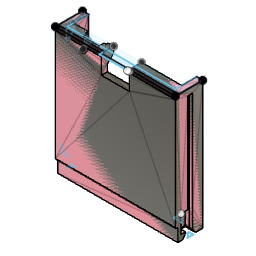
MicrocontrollerHousing (Autodesk Fusion 360 design; units mm, degrees)
Autodesk Fusion 360 part; units mm, degrees
sketch "Sketch1" plane through (0, 0, 0) normal (0, 0, 1) x (1, 0, 0)
ref_plane "WorkPlane1" through (0, 0, 0) normal (0, 0, 1) x (1, 0, 0)
sketch "Sketch2" plane through (0, 0, 0) normal (0, 0, 1) x (1, 0, 0)
  line L0 (-0.0018, 6.8149) -> (30, 6.8149)
  line L1 (30, 6.8149) -> (30, 0)
  line L2 (30, 0) -> (-0.0018, 0)
  line L3 (-0.0018, 0) -> (-0.0018, 6.8149)
  line L4 (14.9991, 3.4075) -> (25.7991, 3.4075)
  line L5 (14.9991, 3.4075) -> (4.1991, 3.4075)
  line L6 (14.9991, 4.3075) -> (4.6991, 4.3075)
  line L7 (14.9991, 4.3075) -> (25.2991, 4.3075)
  line L8 (14.9991, 2.5075) -> (4.6991, 2.5075)
  line L9 (14.9991, 2.5075) -> (25.2991, 2.5075)
  line L10 (14.9991, 4.3075) -> (25.2991, 4.3075)
  line L11 (14.9991, 4.3075) -> (4.6991, 4.3075)
  line L12 (25.7991, 3.8075) -> (25.7991, 3.4075)
  line L13 (4.1991, 3.0075) -> (4.1991, 3.4075)
  line L14 (4.1991, 3.8075) -> (4.1991, 3.4075)
  line L15 (25.7991, 3.4075) -> (25.7991, 3.0075)
  arc A0 (4.6991, 4.3075) -> (4.1991, 3.8075) centre (4.6991, 3.8075) ccw
  arc A1 (4.1991, 3.0075) -> (4.6991, 2.5075) centre (4.6991, 3.0075) ccw
  arc A2 (25.2991, 2.5075) -> (25.7991, 3.0075) centre (25.2991, 3.0075) ccw
  arc A3 (25.7991, 3.8075) -> (25.2991, 4.3075) centre (25.2991, 3.8075) ccw
  line L16 (14.9991, 3.4075) -> (14.9995, 3.4074)
  line L17 (15, 3.4075) -> (14.9995, 3.4074)
  dimension "d2" = 10.8
  dimension "d3" = 10.8
  dimension "d8" = 0.5
  constraint horizontal L0
  constraint vertical L1
  constraint horizontal L2
  constraint vertical L3
  constraint parallel L2 L4
  constraint parallel L4 L5
  constraint perpendicular L4 L12
  constraint perpendicular L5 L13
  constraint perpendicular L5 L14
  constraint parallel L5 L6
  constraint parallel L4 L7
  constraint tangent L14 A0
  constraint tangent L6 A0
  constraint parallel L5 L8
  constraint tangent L13 A1
  constraint tangent L8 A1
  constraint equal A0 A1
  constraint parallel L4 L9
  constraint tangent L9 A2
  constraint tangent L15 A2
  constraint equal A0 A2
  constraint tangent L12 A3
  constraint tangent L7 A3
  constraint equal A0 A3
  constraint parallel L4 L10
  constraint parallel L5 L11
  constraint coincident L4 L17.start
  measures "d2" distance of L4.start L4.end
  measures "d3" distance of L4.start L5.end
  measures "d8" radius of A0
sketch "Sketch4" plane through (0, 0, 0) normal (1, 0, 0) x (0, 1, 0)
  line L0 (6.8002, -0.0004) -> (6.8002, 32)
  line L1 (6.8002, 32) -> (0.8415, 32)
  line L2 (6.8002, -0.0004) -> (-0.2407, -0.0004)
  line L3 (-0.0066, 3.4989) -> (-0.0585, 31.0983)
  line L4 (4.9902, -0.0004) -> (4.2999, 0.9325)
  line L5 (4.2999, 0.9325) -> (4.25, 0.9325)
  line L6 (4.25, 0.9325) -> (4.25, 4.0597)
  line L7 (4.25, 4.0597) -> (2.5001, 4.0597)
  line L8 (2.5001, 1.39) -> (2.5001, 0.9325)
  line L9 (2.5001, 0.9325) -> (2.4506, 0.9325)
  line L10 (2.4506, 0.9325) -> (1.7589, -0.0004)
  line L11 (2.5001, 1.39) -> (1.4001, 1.39)
  line L12 (1.4001, 1.39) -> (1.4001, 5.86)
  line L13 (1.4001, 5.86) -> (3.0784, 5.86)
  line L14 (3.0784, 5.86) -> (3.0784, 30.5)
  line L15 (3.0784, 30.5) -> (4.25, 30.5)
  line L16 (4.25, 30.5) -> (4.25, 4.0597)
  line L17 (0.5999, -0.0004) -> (0.5999, 3.2)
  line L18 (0.5999, 3.2) -> (0.294, 3.1994)
  arc A0 (0.8415, 32) -> (-0.0585, 31.0983) centre (0.8415, 31.1) ccw
  arc A1 (-0.0066, 3.4989) -> (0.294, 3.1994) centre (0.2934, 3.4994) ccw
  line L19 (2.5001, 4.0597) -> (1.4001, 4.0597)
  dimension "d9" = 0.9
  dimension "d10" = 0.3
  constraint vertical L0
  constraint perpendicular L0 L1
  constraint perpendicular L0 L2
  constraint coincident L2 L4.start
  constraint parallel L2 L5
  constraint perpendicular L5 L6
  constraint perpendicular L6 L7
  constraint perpendicular L7 L8
  constraint perpendicular L8 L9
  constraint coincident L2 L10.end
  constraint perpendicular L8 L11
  constraint perpendicular L11 L12
  constraint perpendicular L12 L13
  constraint perpendicular L13 L14
  constraint perpendicular L14 L15
  constraint coincident L2 L17.start
  constraint perpendicular L2 L17
  constraint perpendicular L3 L18
  constraint tangent L1 A0
  constraint tangent L3 A0
  constraint tangent L18 A1
  constraint tangent L3 A1
  constraint coincident L12 L19.end
  constraint perpendicular L12 L19
  measures "d9" radius of A0
  measures "d10" radius of A1
ref_plane "WorkPlane2" through (14.9991, 3.4075, 32) normal (0, 0, 1) x (1, 0, 0)
sketch "Sketch5" plane through (14.9991, 3.4075, 32) normal (0, 0, 1) x (1, 0, 0)
  line L0 (-14.9991, 3.3927) -> (-14.9991, -3.4075)
  line L1 (-14.9991, -3.4075) -> (15.0009, -3.4075)
  line L2 (15.0009, -3.4075) -> (15.0009, 3.4075)
  line L3 (13.5009, 3.3927) -> (13.5009, 3.4067)
  line L4 (13.5009, 3.3927) -> (13.5009, -1.9074)
  line L5 (13.5009, -1.9074) -> (-13.4991, -1.9074)
  line L6 (-13.4991, -1.9074) -> (-13.5017, 3.3934)
  line L7 (15.0009, 3.4075) -> (13.5009, 3.4067)
  line L8 (-13.5017, 3.3934) -> (-14.9991, 3.3927)
  point P0 (-14.9991, 3.3927)
  point P1 (-14.9991, -3.4075)
  point P2 (15.0009, -3.4075)
  point P3 (15.0009, 3.4075)
  constraint coincident P0 L0.start
  constraint coincident P1 L0.end
  constraint coincident P2 L1.end
  constraint coincident P3 L2.end
  constraint perpendicular L3 L7
  constraint perpendicular L1 L4
  constraint perpendicular L4 L5
  constraint coincident L6.end L7
  constraint perpendicular L6 L7
  constraint collinear L7 L8
extrude "Extrude1" add sketch "Sketch5" against normal blind 32
extrude "Extrude2" add sketch "Sketch2" along normal blind 2
sketch "Side Slats" plane through (0, 0, 0) normal (0, 0, 1) x (1, 0, 0)
  line L0 (29.9999, 3.0777) -> (29.19, 3.93)
  line L1 (29.19, 3.93) -> (29.19, 4.25)
  line L2 (29.19, 4.25) -> (30, 4.25)
  line L3 (-0.0001, 3.0776) -> (0.81, 3.93)
  line L4 (0.81, 3.93) -> (0.81, 4.25)
  line L5 (0.81, 4.25) -> (0, 4.25)
  line L6 (-0.0001, 3.0776) -> (-0.201, 2.8662)
  line L7 (-0.201, 2.8662) -> (-0.2009, 4.25)
  line L8 (0, 4.25) -> (-0.2009, 4.25)
  line L9 (30, 4.25) -> (30.168, 4.25)
  line L10 (29.9999, 3.0777) -> (30.168, 2.9008)
  line L11 (30.168, 2.9008) -> (30.168, 4.25)
  constraint vertical L1
  constraint perpendicular L1 L2
  constraint vertical L4
  constraint perpendicular L4 L5
  constraint parallel L3 L6
  constraint perpendicular L7 L8
  constraint parallel L0 L10
  constraint perpendicular L9 L11
extrude "Extrude16" cut sketch "Side Slats" along normal blind 30.5
sketch "Sketch7" plane through (0, 0, 0) normal (1, 0, 0) x (0, 1, 0)
extrude "Extrude4" cut sketch "Sketch4" along normal blind 1.8 contours L2 L4 L5 L6 L7 L8 L9 L10 L11 L12 L19
extrude "Extrude5" cut sketch "Sketch4" against normal blind 1.2 contours L2 L4 L5 L6 L7 L8 L9 L10 L11 L12 L19
ref_plane "WorkPlane3" through (30, 0, 0) normal (1, 0, 0) x (0, 1, 0)
sketch "Sketch8" plane through (30, 0, 0) normal (1, 0, 0) x (0, 1, 0)
  line L0 (1.76, 0) -> (2.4501, 0.9324)
  line L1 (2.4501, 0.9324) -> (2.5001, 0.9324)
  line L2 (2.5001, 0.9324) -> (2.5001, 1.3897)
  line L3 (2.5001, 4.0595) -> (4.25, 4.0602)
  line L4 (4.25, 4.0602) -> (4.25, 0.9324)
  line L5 (4.25, 0.9324) -> (4.3, 0.9324)
  line L6 (4.3, 0.9324) -> (4.9902, -0.0001)
  line L7 (4.9902, -0.0001) -> (1.76, 0)
  line L8 (2.5001, 1.3897) -> (1.4001, 1.3897)
  line L9 (1.4001, 1.3897) -> (1.4001, 4.06)
  line L10 (1.4001, 4.06) -> (2.5001, 4.0595)
  constraint horizontal L1
  constraint perpendicular L1 L2
  constraint perpendicular L1 L4
  constraint perpendicular L4 L5
  constraint perpendicular L2 L8
  constraint perpendicular L8 L9
extrude "Extrude6" cut sketch "Sketch8" against normal blind 1.8
ref_plane "WorkPlane4" through (0, 0, 1.5) normal (0, 0, 1) x (1, 0, 0)
sketch "Sketch9" plane through (0, 0, 1.5) normal (0, 0, 1) x (1, 0, 0)
  line L0 (1.5, 5.3) -> (2.5, 5.3)
  line L1 (2.5, 5.3) -> (2.5, 1.5)
  line L2 (2.5, 1.5) -> (1.5, 1.5)
  line L3 (28.5, 5.3) -> (27.5, 5.3)
  line L4 (27.5, 5.3) -> (27.5, 1.5001)
  line L5 (27.5, 1.5001) -> (28.5, 1.5001)
  line L6 (1.6305, 5.3) -> (1.4386, 5.3)
  line L7 (1.4386, 5.3) -> (1.4386, 1.5)
  line L8 (1.4386, 1.5) -> (1.5958, 1.5)
  line L9 (28.4487, 5.3) -> (28.5452, 5.3)
  line L10 (28.5452, 5.3) -> (28.5453, 1.5001)
  line L11 (28.4238, 1.5001) -> (28.5453, 1.5001)
  constraint horizontal L0
  constraint perpendicular L0 L1
  constraint perpendicular L1 L2
  constraint horizontal L3
  constraint perpendicular L3 L4
  constraint perpendicular L4 L5
  constraint coincident L0 L6.start
  constraint parallel L0 L6
  constraint perpendicular L2 L7
  constraint coincident L2 L8.end
  constraint parallel L2 L8
  constraint coincident L3 L9.start
  constraint perpendicular L9 L10
  constraint coincident L5 L11.start
  constraint perpendicular L10 L11
extrude "Extrude7" add sketch "Sketch9" along normal blind 4 contours L0 L1 L2 L6 L7 L8
extrude "Extrude8" add sketch "Sketch9" along normal blind 4 contours L3 L4 L5 L9 L10 L11
ref_plane "WorkPlane5" through (0, 6, 0) normal (0, 1, 0) x (0, 0, 1)
sketch "Sketch10" plane through (0, 6, 0) normal (0, 1, 0) x (1, 0, 0)
  line L0 (2.5, -4.5) -> (1.5001, -5.5)
  line L1 (1.5001, -5.5) -> (2.5, -5.5)
  line L2 (2.5, -5.5) -> (2.5, -4.5)
  line L3 (28.5, -5.5) -> (27.5, -5.5)
  line L4 (27.5, -5.5) -> (27.5, -4.5)
  line L5 (27.5, -4.5) -> (28.5, -5.5)
  constraint horizontal L1
  constraint perpendicular L1 L2
  constraint perpendicular L2 L3
  constraint perpendicular L3 L4
extrude "Extrude9" cut sketch "Sketch10" against normal blind 4.5
extrude "Extrude10" cut sketch "Sketch8" against normal blind 1.8
extrude "Extrude11" cut sketch "Sketch4" along normal blind 1.8 contours L2 L4 L5 L6 L7 L8 L9 L10 L11 L12 L19
sketch "Sketch11" plane through (30, 0, 0) normal (1, 0, 0) x (0, 1, 0)
  line L0 (1.76, 0) -> (2.4501, 0.9324)
  line L1 (2.4501, 0.9324) -> (2.5001, 0.9324)
  line L2 (2.5001, 0.9324) -> (2.5001, 1.3897)
  line L3 (2.5001, 1.3897) -> (1.4001, 1.3897)
  line L4 (1.4001, 1.3897) -> (1.4001, 4.06)
  line L5 (1.4001, 4.06) -> (2.5001, 4.0595)
  line L6 (2.5001, 4.0595) -> (3.0776, 4.0597)
  line L7 (6.8149, 32) -> (0, 32)
  line L8 (0, 32) -> (0, 0)
  line L9 (4.9901, 0) -> (6.8149, 0)
  line L10 (0.6001, 0) -> (0.012, 0)
  line L11 (0.012, 3.1995) -> (0.6001, 3.1995)
  line L12 (0.6001, 3.1995) -> (0.6001, 0)
  line L13 (0.0679, 0) -> (-0.3097, 0)
  line L14 (-0.3097, 0) -> (-0.3097, 3.1995)
  line L15 (0.0854, 3.1995) -> (-0.3097, 3.1995)
  line L16 (0, 3.5529) -> (0, 3.1995)
  line L17 (0.6001, 3.1408) -> (0.6001, 3.6309)
  line L18 (0.6001, 3.6309) -> (0, 3.6309)
  line L19 (0, 3.5218) -> (0, 3.6309)
  line L20 (3.0776, 4.0597) -> (3.0776, 30.5)
  line L21 (3.0776, 30.5) -> (4.25, 30.5)
  line L22 (4.25, 30.5) -> (4.25, 0.9324)
  line L23 (4.25, 0.9324) -> (4.3, 0.9324)
  line L24 (4.3, 0.9324) -> (4.9901, 0)
  line L25 (6.8149, 0) -> (6.8149, 2)
  line L26 (6.8149, 2) -> (6.8149, 32)
  line L27 (0, 0) -> (1.76, 0)
  constraint horizontal L10
  constraint horizontal L11
  constraint vertical L12
  constraint coincident L9 L10.start
  constraint coincident L10 L13.start
  constraint perpendicular L13 L14
  constraint coincident L11 L15.start
  constraint perpendicular L14 L15
  constraint coincident L8 L16.start
  constraint coincident L15 L16.end
  constraint coincident L8 L16.end
  constraint perpendicular L15 L16
  constraint coincident L12 L17.start
  constraint perpendicular L11 L17
  constraint coincident L8 L18.end
  constraint perpendicular L8 L18
  constraint coincident L16 L19.start
extrude "Extrude12" cut sketch "Sketch11" against normal through all contours L8 L10 L11 L12 L13 L15 L17 L27 | L8 L13 L14 L15
sketch "Sketch12" plane through (30, 0, 0) normal (1, 0, 0) x (0, 1, 0)
  line L0 (0.6001, 3.1995) -> (0.6001, 0)
  line L1 (0.6001, 0) -> (1.76, 0)
  line L2 (1.76, 0) -> (2.4501, 0.9324)
  line L3 (2.4501, 0.9324) -> (2.5001, 0.9324)
  line L4 (2.5001, 0.9324) -> (2.5001, 1.3897)
  line L5 (2.5001, 1.3897) -> (1.4001, 1.3897)
  line L6 (1.4001, 1.3897) -> (1.4001, 4.06)
  line L7 (1.4001, 4.06) -> (2.5001, 4.0595)
  line L8 (2.5001, 4.0595) -> (3.0776, 4.0597)
  line L9 (6.8149, 32) -> (0, 32)
  line L10 (0, 32) -> (0, 3.1995)
  line L11 (0, 3.1995) -> (0.6001, 3.1995)
  line L12 (0, 3.4998) -> (0.716, 3.4998)
  line L13 (0.6001, 3.1995) -> (0.6001, 3.4998)
  line L14 (0, 3.4998) -> (0, 3.4995)
  line L15 (0.6001, 3.1995) -> (0.3, 3.1995)
  arc A0 (0, 3.4995) -> (0.3, 3.1995) centre (0.3, 3.4995) ccw
  line L16 (3.0776, 4.0597) -> (3.0776, 30.5)
  line L17 (3.0776, 30.5) -> (4.25, 30.5)
  line L18 (4.25, 30.5) -> (4.25, 0.9324)
  line L19 (4.25, 0.9324) -> (4.3, 0.9324)
  line L20 (4.3, 0.9324) -> (4.9901, 0)
  line L21 (4.9901, 0) -> (6.8149, 0)
  line L22 (6.8149, 0) -> (6.8149, 2)
  line L23 (6.8149, 2) -> (6.8149, 32)
  dimension "d37" = 0.3
  constraint coincident L10 L12.start
  constraint perpendicular L10 L12
  constraint coincident L0.start L11.end
  constraint coincident L12 L13.end
  constraint perpendicular L12 L13
  constraint tangent L15 A0
  constraint tangent L14 A0
  measures "d37" radius of A0
extrude "Extrude13" cut sketch "Sketch12" against normal through all contours L10 L11 A0
sketch "Sketch13" plane through (0, 0, 0) normal (0, 0, -1) x (1, 0, 0)
  line L0 (25.7991, -3.0075) -> (25.7991, -3.8075)
  arc A0 (25.2991, -4.3075) -> (25.7991, -3.8075) centre (25.2991, -3.8075) ccw
  line L1 (25.2991, -4.3075) -> (4.6991, -4.3075)
  arc A1 (4.1991, -3.8075) -> (4.6991, -4.3075) centre (4.6991, -3.8075) ccw
  line L2 (4.1991, -3.8075) -> (4.1991, -3.0075)
  arc A2 (4.6991, -2.5075) -> (4.1991, -3.0075) centre (4.6991, -3.0075) ccw
  line L3 (4.6991, -2.5075) -> (25.2991, -2.5075)
  arc A3 (25.7991, -3.0075) -> (25.2991, -2.5075) centre (25.2991, -3.0075) ccw
  line L4 (30, -0.6001) -> (-0.0018, -0.6001)
  line L5 (-0.0018, -0.6001) -> (-0.0018, -1.7592)
  line L6 (-0.0018, -1.7592) -> (1.8, -1.7592)
  line L7 (1.8, -1.7592) -> (1.8, -4.9899)
  line L8 (1.8, -4.9899) -> (-0.0018, -4.9899)
  line L9 (-0.0018, -4.9899) -> (-0.0018, -6.8149)
  line L10 (-0.0018, -6.8149) -> (30, -6.8149)
  line L11 (30, -6.8149) -> (30, -4.9901)
  line L12 (30, -4.9901) -> (28.2, -4.9901)
  line L13 (28.2, -4.9901) -> (28.2, -1.76)
  line L14 (28.2, -1.76) -> (30, -1.76)
  line L15 (30, -1.76) -> (30, -0.6001)
  line L16 (14.6109, -2.2) -> (17.9456, -2.2)
  line L17 (19.2456, -3.5) -> (19.2456, -3.5306)
  line L18 (17.9456, -4.8306) -> (14.6109, -4.8306)
  line L19 (14.6109, -2.2) -> (12.0539, -2.2)
  line L20 (10.7539, -3.5) -> (10.7539, -3.5306)
  line L21 (12.0539, -4.8306) -> (14.6109, -4.8306)
  arc A4 (12.0539, -2.2) -> (10.7539, -3.5) centre (12.0539, -3.5) ccw
  arc A5 (10.7539, -3.5306) -> (12.0539, -4.8306) centre (12.0539, -3.5306) ccw
  arc A6 (19.2456, -3.5) -> (17.9456, -2.2) centre (17.9456, -3.5) ccw
  arc A7 (17.9456, -4.8306) -> (19.2456, -3.5306) centre (17.9456, -3.5306) ccw
  dimension "d39" = 1.3
  dimension "d40" = 1.3
  dimension "d41" = 1.3
  dimension "d42" = 1.3
  constraint horizontal L16
  constraint vertical L17
  constraint horizontal L18
  constraint horizontal L19
  constraint vertical L20
  constraint horizontal L21
  constraint tangent L20 A4
  constraint tangent L19 A4
  constraint tangent L20 A5
  constraint tangent L21 A5
  constraint tangent L16 A6
  constraint tangent L17 A6
  constraint tangent L17 A7
  constraint tangent L18 A7
  measures "d39" radius of A4
  measures "d40" radius of A5
  measures "d41" radius of A6
  measures "d42" radius of A7
extrude "Extrude14" add sketch "Sketch13" against normal blind 2 contours L0 A0 L1 L3 A3 L17 A6 A7 | L1 L3 L17 L20 A4 A5 A6 A7 | L1 A1 L2 A2 L3 L20 A4 A5
extrude "Extrude15" cut sketch "Sketch13" against normal through all contours L1 L3 L17 L20 A4 A5 A6 A7 | L3 L16 L19 A4 A6 | L1 L18 L21 A5 A7
sketch "Sketch14" plane through (30, 0, 0) normal (1, 0, 0) x (0, 1, 0)
  arc A0 (0, 3.4995) -> (0.3, 3.1995) centre (0.3, 3.4995) ccw
  line L0 (0.3, 3.1995) -> (0.6001, 3.1995)
  line L1 (0.6001, 3.1995) -> (0.6001, 0)
  line L2 (0.6001, 0) -> (1.76, 0)
  line L3 (1.76, 0) -> (2.4501, 0.9324)
  line L4 (2.4501, 0.9324) -> (2.5001, 0.9324)
  line L5 (2.5001, 0.9324) -> (2.5001, 1.3897)
  line L6 (2.5001, 1.3897) -> (1.4001, 1.3897)
  line L7 (1.4001, 1.3897) -> (1.4001, 4.06)
  line L8 (1.4001, 4.06) -> (2.5001, 4.0595)
  line L9 (2.5001, 4.0595) -> (3.0776, 4.0597)
  line L10 (3.0776, 4.0597) -> (3.0776, 30.5)
  line L11 (3.0776, 30.5) -> (4.25, 30.5)
  line L12 (4.25, 30.5) -> (4.25, 0.9324)
  line L13 (4.25, 0.9324) -> (4.3, 0.9324)
  line L14 (4.3, 0.9324) -> (4.9901, 0)
  line L15 (4.9901, 0) -> (6.8149, 0)
  line L16 (6.8149, 0) -> (6.8149, 2)
  line L17 (6.8149, 2) -> (6.8149, 32)
  line L18 (6.8149, 32) -> (0, 32)
  line L19 (0, 32) -> (0, 3.4995)
  line L20 (0.8001, 32) -> (0.8, 32)
  line L21 (0, 31.2) -> (0, 31.2001)
  line L22 (0, 31.2001) -> (0.8001, 31.2001)
  line L23 (0.8001, 31.2001) -> (0.8001, 32)
  arc A1 (0.8, 32) -> (0, 31.2) centre (0.8, 31.2) ccw
  dimension "d48" = 0.8
  constraint horizontal L20
  constraint vertical L21
  constraint horizontal L22
  constraint vertical L23
  constraint coincident L19 L21.end
  constraint coincident L18 L20.start
  constraint tangent L21 A1
  constraint tangent L20 A1
  measures "d48" radius of A1
extrude "Extrude17" cut sketch "Sketch14" against normal through all contours L18 L19 A1
ref_plane "WorkPlane6" through (0, 1.4, 0) normal (0, 1, 0) x (0, 0, 1)
sketch "Sketch15" plane through (0, 1.4, 0) normal (0, 1, 0) x (1, 0, 0)
  line L0 (1.8, -4.0597) -> (0, -5.8599)
  line L1 (0, -5.8599) -> (0, -4.0597)
  line L2 (0, -4.0597) -> (1.8, -4.0597)
  line L3 (28.2005, -4.0596) -> (30, -5.8599)
  line L4 (30.0677, -4.0596) -> (30.0677, -5.9277)
  line L5 (29.9608, -5.8208) -> (30.0677, -5.9277)
  line L6 (30.0677, -4.0596) -> (30.0677, -3.9862)
  line L7 (30.0677, -3.9862) -> (28.2005, -3.9862)
  line L8 (28.2005, -4.0596) -> (28.2005, -3.9862)
  constraint vertical L1
  constraint perpendicular L1 L2
  constraint coincident L3 L5.start
  constraint parallel L3 L5
  constraint perpendicular L6 L7
  constraint perpendicular L7 L8
extrude "Extrude18" cut sketch "Sketch15" along normal blind 2.85 contours L0 L1 L2
extrude "Extrude19" cut sketch "Sketch15" along normal blind 2.85 contours L3 L4 L5 L6 L7 L8
ref_plane "WorkPlane7" through (0, 5, 0) normal (0, 1, 0) x (0, 0, 1)
sketch "Sketch16" plane through (0, 5, 0) normal (0, 1, 0) x (1, 0, 0)
sketch "Sketch17" plane through (0, 4.25, 0) normal (0, -1, 0) x (1, 0, 0)
  line L0 (0.81, 5.0499) -> (0, 5.8599)
  line L1 (0, 5.8599) -> (0, 4.0597)
  line L2 (0, 4.0597) -> (0, 2)
  line L3 (0, 2) -> (-0.0018, 2)
  line L4 (-0.0018, 2) -> (-0.0018, 0.9325)
  line L5 (-0.0018, 0.9325) -> (1.8, 0.9325)
  line L6 (1.8, 0.9325) -> (1.8, 4.0597)
  line L7 (1.8, 4.0597) -> (0.81, 5.0499)
  line L8 (-0.0018, 0.9325) -> (0.0499, 0.9999)
  line L9 (0.0499, 0.9999) -> (1.8, 0.9999)
  line L10 (1.8, 0.9325) -> (-0.0018, 0.9325)
  line L11 (0.0499, 0.9999) -> (-0.0018, 0.9999)
  line L12 (-0.0018, 0.9325) -> (-0.0018, 0.9999)
  constraint coincident L4.end L5.start
  constraint coincident L6 L9.end
  constraint perpendicular L6 L9
  constraint coincident L5.end L6.start
  constraint coincident L4 L11.end
  constraint perpendicular L4 L11
fillet "Fillet1" radius 0.07 1 edges at (0.8991, 4.25, 0.9325)
extrude "Extrude20" add sketch "Sketch17" against normal blind 0.05 contours L4 L8 L11 L12
sketch "Sketch18" plane through (0, 2.5001, 0) normal (0, 1, 0) x (-1, 0, 0)
  line L0 (-1.8, 0.9325) -> (0.0018, 0.9325)
  line L1 (0.0018, 0.9325) -> (0.0018, 1.39)
  line L2 (0.0018, 1.39) -> (-1.8, 1.39)
  line L3 (-1.8, 1.39) -> (-1.8, 0.9325)
  line L4 (-1.8, 0.9325) -> (0.0018, 0.9325)
  line L5 (0.0018, 0.9325) -> (-0.05, 0.9999)
  line L6 (-0.05, 0.9999) -> (-1.8, 0.9999)
  line L7 (-1.8, 0.9325) -> (0.0018, 0.9325)
  line L8 (-0.05, 0.9999) -> (0.0018, 0.9999)
  line L9 (0.0018, 0.9325) -> (0.0018, 0.9999)
  constraint coincident L0.start L3.end
  constraint coincident L0.end L1.start
  constraint coincident L3 L6.end
  constraint perpendicular L3 L6
  constraint coincident L1 L8.end
  constraint perpendicular L1 L8
fillet "Fillet2" radius 0.075 1 edges at (0.8991, 2.5001, 0.9325)
extrude "Extrude21" add sketch "Sketch18" against normal blind 0.07 contours L1 L5 L8 L9
sketch "Sketch19" plane through (0, 4.25, 0) normal (0, -1, 0) x (1, 0, 0)
  line L0 (29.19, 0.9324) -> (30, 0.9324)
  line L1 (30, 0.9324) -> (30, 30.5)
  line L2 (30, 30.5) -> (29.19, 30.5)
  line L3 (29.19, 30.5) -> (29.19, 0.9324)
  line L4 (30, 0.9324) -> (29.9497, 0.9999)
  line L5 (29.9497, 0.9999) -> (28.1999, 0.9999)
  line L6 (28.1999, 0.9999) -> (28.1999, 0.9324)
  line L7 (28.1999, 0.9324) -> (30, 0.9324)
  line L8 (29.9497, 0.9999) -> (30, 0.9999)
  line L9 (30, 0.9324) -> (30, 0.9999)
  constraint coincident L0.end L1.start
  constraint perpendicular L1 L5
  constraint perpendicular L5 L6
  constraint perpendicular L1 L7
  constraint coincident L1 L8.end
  constraint perpendicular L1 L8
fillet "Fillet3" radius 0.07 2 edges at (29.595, 4.25, 0.9324) (28.695, 4.25, 0.9324)
extrude "Extrude22" add sketch "Sketch19" against normal blind 0.06 contours L1 L4 L8 L9
sketch "Sketch20" plane through (0, 2.5001, 0) normal (0, 1, 0) x (-1, 0, 0)
  line L0 (-30, 1.3897) -> (-30, 0.9324)
  line L1 (-30, 0.9324) -> (-28.2, 0.9324)
  line L2 (-28.2, 0.9324) -> (-28.2, 1.3897)
  line L3 (-28.2, 1.3897) -> (-30, 1.3897)
  line L4 (-28.2, 0.9324) -> (-30, 0.9324)
  line L5 (-30, 0.9324) -> (-29.9501, 1)
  line L6 (-29.9501, 1) -> (-28.2, 1)
  line L7 (-28.2, 0.9324) -> (-28.2, 1)
  line L8 (-29.9501, 1) -> (-30, 1)
  constraint coincident L1.end L2.start
  constraint coincident L0.end L1.start
  constraint coincident L2 L6.end
  constraint perpendicular L2 L6
  constraint coincident L0 L8.end
  constraint perpendicular L0 L8
fillet "Fillet4" radius 0.075 1 edges at (29.1, 2.5001, 0.9324)
extrude "Extrude23" add sketch "Sketch20" against normal blind 0.1 contours L0 L5 L8
chamfer "Chamfer1" distance 0.74 distance2 1 1 edges at (1.8, 3.3745, 0) measured on face at (4.7846, 3.4163, 0)
chamfer "Chamfer2" distance 0.74 distance2 1 1 edges at (28.2, 3.375, 0) measured on face at (25.2152, 3.4167, 0)
sketch "Sketch21" plane through (0, 0, 2) normal (0, 0, 1) x (-1, 0, 0)
  arc A0 (-19.2456, -3.5306) -> (-17.9456, -4.8306) centre (-17.9456, -3.5306) ccw
  line L0 (-19.2456, -3.5306) -> (-19.2456, -3.5)
  arc A1 (-17.9456, -2.2) -> (-19.2456, -3.5) centre (-17.9456, -3.5) ccw
  line L1 (-17.9456, -2.2) -> (-12.0539, -2.2)
  arc A2 (-10.7539, -3.5) -> (-12.0539, -2.2) centre (-12.0539, -3.5) ccw
  line L2 (-10.7539, -3.5) -> (-10.7539, -3.5306)
  arc A3 (-12.0539, -4.8306) -> (-10.7539, -3.5306) centre (-12.0539, -3.5306) ccw
  line L3 (-12.0539, -4.8306) -> (-17.9456, -4.8306)
  line L4 (-28.4487, -5.3) -> (-28.5, -5.3)
  line L5 (-28.5, -5.3) -> (-28.5, -6.8002)
  line L6 (-28.5, -6.8002) -> (-28.5, -6.8142)
  line L7 (-28.5, -6.8142) -> (-30, -6.8149)
  line L8 (-30, -6.8149) -> (0.0018, -6.8149)
  line L9 (0.0018, -6.8149) -> (0.0018, -4.25)
  line L10 (0.0018, -4.25) -> (0, -4.25)
  line L11 (0, -4.25) -> (0, -6.8002)
  line L12 (0, -6.8002) -> (-1.4974, -6.8009)
  line L13 (-1.4974, -6.8009) -> (-1.4981, -5.3)
  line L14 (-1.4981, -5.3) -> (-2.5, -5.3)
  line L15 (-2.5, -5.3) -> (-2.5, -1.5001)
  line L16 (-2.5, -1.5001) -> (-27.5, -1.5001)
  line L17 (-27.5, -1.5001) -> (-27.5, -5.3)
  line L18 (-27.5, -5.3) -> (-28.4487, -5.3)
extrude "Extrude24" cut sketch "Sketch21" against normal blind 0.5 contours L4 L5 L6 L7 L8 L9 L10 L11 L12 L13 L14 L15 L16 L17 L18
chamfer "Chamfer3" distance 1.4 distance2 0.37 8 edges at (14.9997, 2.2, 1.5) (18.8648, 2.5807, 1.5) (19.2456, 3.5153, 1.5) (18.8648, 4.4498, 1.5) (14.9997, 4.8306, 1.5) (11.1347, 4.4498, 1.5) (10.7539, 3.5153, 1.5) (11.1347, 2.5807, 1.5) measured on face at (14.0178, 2.2, 0.5) measured on face at (18.4287, 2.2931, 1) measured on face at (19.2456, 3.5204, 1) measured on face at (18.1916, 4.8071, 0.5) measured on face at (14.0178, 4.8306, 0.5) measured on face at (11.1568, 4.4714, 1) measured on face at (10.7539, 3.5102, 0.5) measured on face at (11.9921, 2.2014, 0.5)
other "Base Mesh Feature3"
sketch "Sketch22" plane through (0, 0, 0) normal (0, 0, -1) x (1, 0, 0)
  line L0 (27.46, -1.76) -> (30, -1.76)
  line L1 (30, -1.76) -> (30, -0.6001)
  line L2 (30, -0.6001) -> (-0.0018, -0.6001)
  line L3 (-0.0018, -0.6001) -> (-0.0018, -1.7592)
  line L4 (-0.0018, -1.7592) -> (2.54, -1.7592)
  line L5 (2.54, -1.7592) -> (2.54, -4.9899)
  line L6 (2.54, -4.9899) -> (-0.0018, -4.9899)
  line L7 (-0.0018, -4.9899) -> (-0.0018, -6.8149)
  line L8 (-0.0018, -6.8149) -> (30, -6.8149)
  line L9 (30, -6.8149) -> (30, -4.9901)
  line L10 (30, -4.9901) -> (27.46, -4.9901)
  line L11 (27.46, -4.9901) -> (27.46, -1.76)
  arc A0 (17.9456, -4.8306) -> (19.2456, -3.5306) centre (17.9456, -3.5306) ccw
  line L12 (17.9456, -4.8306) -> (12.0539, -4.8306)
  arc A1 (10.7539, -3.5306) -> (12.0539, -4.8306) centre (12.0539, -3.5306) ccw
  line L13 (10.7539, -3.5306) -> (10.7539, -3.5)
  arc A2 (12.0539, -2.2) -> (10.7539, -3.5) centre (12.0539, -3.5) ccw
  line L14 (12.0539, -2.2) -> (17.9456, -2.2)
  arc A3 (19.2456, -3.5) -> (17.9456, -2.2) centre (17.9456, -3.5) ccw
  line L15 (19.2456, -3.5) -> (19.2456, -3.5306)
  line L16 (10.7539, -3.5) -> (10.7539, -7.316)
  line L17 (10.7539, -7.316) -> (19.2456, -7.316)
  line L18 (19.2456, -3.5) -> (19.2456, -7.316)
  line L19 (19.2456, -3.5) -> (10.7539, -3.5)
  constraint coincident L13.end A2.end
  constraint tangent A2 L16
  constraint perpendicular L13 L17
  constraint coincident A3.start L15.start
  constraint tangent A3 L18
extrude "Extrude25" cut sketch "Sketch22" against normal blind 2.5 contours L8 L16 L17 L18 | L8 A0 L12 A1 L16 L18 | A0 L12 A1 L13 L15 L16 L18 L19
sketch "Sketch23" plane through (0, 1.5001, 0) normal (0, 1, 0) x (-1, 0, 0)
  line L0 (-1.5, 5.5) -> (-1.5, 32)
  line L1 (-1.5, 32) -> (-28.5, 32)
  line L2 (-28.5, 32) -> (-28.5, 5.5)
  line L3 (-28.5, 5.5) -> (-27.5, 5.5)
  line L4 (-27.5, 5.5) -> (-27.5, 4.5)
  line L5 (-27.5, 4.5) -> (-27.5, 4.5)
  line L6 (-27.5, 4.5) -> (-27.5, 2)
  line L7 (-27.5, 2) -> (-2.5, 2)
  line L8 (-2.5, 2) -> (-2.5, 4.5)
  line L9 (-2.5, 4.5) -> (-2.5, 5.5)
  line L10 (-2.5, 5.5) -> (-1.5001, 5.5)
  circle A0 centre (-3.7, 21.5005) radius 0.7502
  circle A1 centre (-3.7, 21.5005) radius 2.2971
  line L11 (-5.3264, 19.874) -> (-5.3243, 19.8761)
  line L12 (-2.0758, 23.1249) -> (-2.0737, 23.127)
  line L13 (-5.3264, 23.1263) -> (-5.3246, 23.1246)
  line L14 (-2.0758, 19.8761) -> (-2.0737, 19.874)
  line L15 (-4.2001, 19.2585) -> (-4.2001, 17.75)
  line L16 (-4.2001, 17.75) -> (-3.2001, 17.75)
  line L17 (-3.2001, 17.75) -> (-3.2001, 19.2584)
  circle A2 centre (-26.3, 21.5) radius 0.7499
  circle A3 centre (-26.3, 21.5) radius 2.3001
  line L18 (-26.8001, 19.255) -> (-26.8001, 17.7501)
  line L19 (-26.8001, 17.7501) -> (-25.8, 17.7501)
  line L20 (-25.8, 17.7501) -> (-25.8, 19.2549)
  constraint perpendicular L11 L13
  constraint concentric A0 A1
  constraint coincident A1 L12.start
  constraint collinear L11 L12
  constraint coincident A0.centre L11
  constraint coincident A1 L11.end
  constraint coincident A1 L13.end
  constraint collinear L13 L14
  constraint coincident A1 L14.start
  constraint coincident A1 L15.start
  constraint vertical L15
  constraint perpendicular L15 L16
  constraint coincident A1 L17.end
  constraint perpendicular L16 L17
  constraint concentric A2 A3
  constraint coincident A3 L18.start
  constraint vertical L18
  constraint perpendicular L18 L19
  constraint coincident A3 L20.end
  constraint perpendicular L19 L20
extrude "Extrude26" add sketch "Sketch23" along normal blind 1.55 contours L0 A1 | A1 L15 L16 L17 | L2 A3 | A3 L18 L19 L20 picked at (-1.9833, 21.5005) picked at (-28.0166, 21.5)
sketch "Sketch24" plane through (25.8, 0, 0) normal (-1, 0, 0) x (0, -1, 0)
  line L0 (-1.5001, 17.7501) -> (-1.5001, 19.2549)
  line L1 (-1.5001, 19.2549) -> (-3.0501, 19.2549)
  line L2 (-3.0501, 19.2549) -> (-3.0501, 17.7501)
  line L3 (-3.0501, 17.7501) -> (-1.5001, 17.7501)
  line L4 (-3.0043, 19.2549) -> (-1.5001, 17.7501)
  line L5 (-3.0501, 17.7501) -> (-3.0501, 17.609)
  line L6 (-3.0501, 17.609) -> (-1.5867, 17.609)
  line L7 (-1.5001, 17.7501) -> (-1.5001, 17.6088)
  line L8 (-1.6673, 17.609) -> (-1.5001, 17.6088)
  constraint coincident L1 L4.start
  constraint coincident L0.start L3.end
  constraint coincident L2.end L3.start
  constraint perpendicular L3 L5
  constraint perpendicular L2 L6
  constraint perpendicular L3 L7
  constraint coincident L6 L8.start
extrude "Extrude27" cut sketch "Sketch24" against normal blind 1.1 contours L1 L2 L3 L4
extrude "Extrude28" cut sketch "Sketch24" along normal blind 23 contours L3 L5 L6 L7 L8 | L1 L2 L3 L4
sketch "Sketch25" plane through (1.5007, 0.0007, 0) normal (1, 0.000492, 0) x (-0.000492, 1, 0)
  line L0 (1.4993, 5.5) -> (5.2992, 5.5)
  line L1 (5.2992, 5.5) -> (5.2992, 1.5)
  line L2 (5.2992, 1.5) -> (6.8002, 1.5)
  line L3 (6.8002, 1.5) -> (6.8002, 32)
  line L4 (6.8002, 32) -> (1.4993, 32)
  line L5 (1.4993, 32) -> (1.4993, 22.1612)
  line L6 (1.4993, 22.1612) -> (1.4993, 20.8398)
  line L7 (1.4993, 20.8398) -> (1.4993, 5.5)
  line L8 (3.0601, 32) -> (3.0488, 30.5)
  line L9 (3.0488, 30.5) -> (1.4993, 28.9501)
  line L10 (1.4993, 28.9501) -> (1.2622, 28.9501)
  line L11 (1.2622, 28.9501) -> (1.2622, 32)
  line L12 (3.0601, 32) -> (1.2622, 32)
  constraint coincident L4 L8.start
  constraint coincident L5 L9.end
  constraint perpendicular L5 L10
  constraint perpendicular L10 L11
  constraint perpendicular L11 L12
extrude "Extrude31" add sketch "Sketch25" along normal blind 27.1 contours L5 L10 L11 L12 | L4 L5 L8 L9 L12
extrude "Extrude29" add sketch "Sketch25" along normal blind 27.1 contours L4 L5 L8 L9 L12
sketch "Sketch26" plane through (0, 0, 32) normal (0, 0, 1) x (-1, 0, 0)
  line L0 (-28.5, -6.8002) -> (-28.5, -3.0741)
  line L1 (-28.5, -3.0741) -> (-1.4992, -3.0608)
  line L2 (-1.4992, -3.0608) -> (-1.4974, -6.8009)
  line L3 (-1.4974, -6.8009) -> (0, -6.8002)
  line L4 (0, -6.8002) -> (0, -0.8)
  line L5 (0, -0.8) -> (-30, -0.8)
  line L6 (-30, -0.8) -> (-30, -6.8149)
  line L7 (-30, -6.8149) -> (-28.5, -6.8142)
  line L8 (-28.5, -6.8142) -> (-28.5, -6.8002)
  line L9 (-11.5, -3.0498) -> (-11.5, -3.0658)
  line L10 (-11.5, -3.0526) -> (-11.5, 0.482)
  line L11 (-11.5, 0.482) -> (-18.9398, 0.482)
  line L12 (-18.5, -3.0431) -> (-18.5, -3.0692)
  line L13 (-18.5, -3.0431) -> (-18.5017, 0.482)
  constraint coincident L1 L9.end
  constraint perpendicular L1 L9
  constraint coincident L9 L10.start
  constraint perpendicular L5 L10
  constraint perpendicular L10 L11
  constraint coincident L1 L12.end
  constraint perpendicular L1 L12
extrude "Extrude30" cut sketch "Sketch26" against normal blind 4.75 contours L1 L5 L9 L10 L12 L13 | L5 L10 L11 L13
sketch "Sketch27" plane through (0, 0, 32) normal (0, 0, 1) x (-1, 0, 0)
  line L0 (-11.5, -0.8) -> (-11.5, -3.0526)
  line L1 (-11.5, -3.0526) -> (-11.5, -3.0658)
  line L2 (-11.5, -3.0658) -> (-1.4992, -3.0608)
  line L3 (-1.4992, -3.0608) -> (-1.4974, -6.8009)
  line L4 (-1.4974, -6.8009) -> (0, -6.8002)
  line L5 (0, -6.8002) -> (0, -0.8)
  line L6 (0, -0.8) -> (-11.5, -0.8)
  line L7 (-5.0966, -2.55) -> (-5.596, -2.5502)
  line L8 (-5.596, -2.5502) -> (-5.5965, -1.35)
  line L9 (-5.5965, -1.35) -> (-9.5961, -1.352)
  line L10 (-9.5961, -1.352) -> (-9.5955, -2.55)
  line L11 (-9.5955, -2.55) -> (-10.0948, -2.5502)
  line L12 (-10.0948, -2.5502) -> (-10.0946, -3.0651)
  line L13 (-5.0966, -2.55) -> (-5.0964, -3.1281)
  line L14 (-5.0964, -3.1281) -> (-10.0945, -3.1306)
  line L15 (-10.0946, -3.0651) -> (-10.0945, -3.1306)
  constraint perpendicular L8 L9
  constraint perpendicular L2 L10
  constraint perpendicular L10 L11
  constraint coincident L2 L12.end
  constraint perpendicular L2 L12
  constraint perpendicular L7 L13
  constraint perpendicular L13 L14
  constraint perpendicular L14 L15
extrude "Extrude32" cut sketch "Sketch27" against normal blind 3 contours L2 L7 L8 L9 L10 L11 L12 L13 | L2 L13 L14 L15
sketch "Sketch28" plane through (5.5972, 0.0028, 0) normal (1, 0.000492, 0) x (-0.000492, 1, 0)
  line L0 (1.5493, 29) -> (2.5475, 29.9985)
  line L1 (2.5475, 29.9985) -> (2.5475, 32)
  line L2 (2.5475, 32) -> (1.3472, 32)
  line L3 (1.3472, 32) -> (1.3472, 29)
  line L4 (1.3472, 29) -> (1.5493, 29)
  line L5 (2.5475, 30.5001) -> (1.3472, 29.3)
  line L6 (1.3472, 29.3) -> (1.3472, 29)
  line L7 (1.5493, 29) -> (1.6956, 29)
  line L8 (1.6956, 29) -> (2.5475, 29.8522)
  line L9 (2.5475, 30.5001) -> (2.5475, 29.8522)
  line L10 (1.5493, 29) -> (1.5493, 29.502)
  constraint coincident L1 L5.start
  constraint coincident L3 L5.end
  constraint coincident L3.end L4.start
  constraint coincident L0.start L4.end
  constraint perpendicular L3 L7
  constraint parallel L0 L8
  constraint parallel L1 L9
  constraint coincident L5 L10.end
  constraint perpendicular L4 L10
extrude "Extrude33" cut sketch "Sketch28" against normal blind 0.5 contours L0 L1 L5 L9 L10 | L0 L7 L8 L9
extrude "Extrude34" cut sketch "Sketch28" along normal blind 4.5 contours L0 L1 L5 L9 L10 | L0 L7 L8 L9
